Autodesk Fusion 360 part; units mm, degrees
(part 20 of 24)
  arc A286 (13.1064, 12.5222) -> (13.1064, 12.5984) centre (13.1064, 12.5603) ccw
  arc A287 (80.518, 13.5509) -> (80.518, 13.6271) centre (80.518, 13.589) ccw
  arc A288 (6.9723, 12.3063) -> (7.0485, 12.3063) centre (7.0104, 12.3063) ccw
  line L141 (7.2644, 10.2743) -> (7.6454, 10.2743)
  line L142 (13.3604, 11.7221) -> (13.3604, 11.1125)
  line L143 (6.1468, 11.1125) -> (7.0104, 11.1125)
  line L144 (6.1468, 11.7221) -> (6.1468, 11.1125)
  line L145 (7.0104, 11.1125) -> (7.0104, 11.7221)
  arc A289 (80.01, 13.4239) -> (80.01, 13.5001) centre (80.01, 13.462) ccw
  arc A290 (80.8101, 13.335) -> (80.7339, 13.335) centre (80.772, 13.335) ccw
  arc A291 (6.9723, 10.5283) -> (7.0485, 10.5283) centre (7.0104, 10.5283) ccw
  arc A292 (7.7724, 12.4714) -> (7.7724, 12.3952) centre (7.7724, 12.4333) ccw
  line L146 (7.7724, 12.4333) -> (12.5984, 12.4333)
  arc A293 (7.0104, 10.5283) -> (7.2644, 10.2743) centre (7.2644, 10.5283) ccw
  arc A294 (7.2644, 10.2362) -> (7.2644, 10.3124) centre (7.2644, 10.2743) ccw
  line L147 (7.0104, 11.7221) -> (6.1468, 11.7221)
  arc A295 (12.6253, 10.4282) -> (12.5715, 10.3744) centre (12.5984, 10.4013) ccw
  line L148 (7.2644, 12.5603) -> (7.6454, 12.5603)
  line L149 (13.1064, 10.2743) -> (12.7254, 10.2743)
  arc A296 (12.5984, 12.3952) -> (12.5984, 12.4714) centre (12.5984, 12.4333) ccw
  arc A297 (13.3985, 10.5283) -> (13.3223, 10.5283) centre (13.3604, 10.5283) ccw
  arc A298 (7.0485, 12.3063) -> (6.9723, 12.3063) centre (7.0104, 12.3063) ccw
  line L150 (12.5984, 12.4333) -> (12.7254, 12.5603)
  arc A299 (13.3985, 12.3063) -> (13.3223, 12.3063) centre (13.3604, 12.3063) ccw
  line L151 (81.5086, 25.0952) -> (81.5086, 25.7048)
  arc A300 (74.3331, 26.289) -> (74.2569, 26.289) centre (74.295, 26.289) ccw
  arc A301 (60.9869, 21.4899) -> (60.9331, 21.4361) centre (60.96, 21.463) ccw
  arc A302 (74.2569, 24.511) -> (74.3331, 24.511) centre (74.295, 24.511) ccw
  arc A303 (75.0301, 26.3891) -> (75.0839, 26.4429) centre (75.057, 26.416) ccw
  arc A304 (74.9569, 26.5699) -> (74.9031, 26.5161) centre (74.93, 26.543) ccw
  arc A305 (74.549, 26.5811) -> (74.549, 26.5049) centre (74.549, 26.543) ccw
  arc A306 (74.93, 24.2189) -> (74.93, 24.2951) centre (74.93, 24.257) ccw
  line L152 (75.057, 26.416) -> (74.93, 26.543)
  arc A307 (80.6069, 26.289) -> (80.6831, 26.289) centre (80.645, 26.289) ccw
  arc A308 (80.6831, 26.289) -> (80.6069, 26.289) centre (80.645, 26.289) ccw
  line L153 (73.4314, 25.7048) -> (73.4314, 25.0952)
  line L154 (80.645, 25.7048) -> (80.645, 25.0952)
  arc A309 (75.0839, 24.3571) -> (75.0301, 24.4109) centre (75.057, 24.384) ccw
  arc A310 (80.0369, 26.5161) -> (79.9831, 26.5699) centre (80.01, 26.543) ccw
  arc A311 (80.391, 26.5049) -> (80.391, 26.5811) centre (80.391, 26.543) ccw
  arc A312 (79.9831, 24.2301) -> (80.0369, 24.2839) centre (80.01, 24.257) ccw
  line L155 (80.391, 26.543) -> (80.01, 26.543)
  arc A313 (80.391, 26.5811) -> (80.391, 26.5049) centre (80.391, 26.543) ccw
  arc A314 (80.391, 24.2951) -> (80.391, 24.2189) centre (80.391, 24.257) ccw
  line L156 (75.057, 24.384) -> (74.93, 24.257)
  arc A315 (74.549, 24.2189) -> (74.549, 24.2951) centre (74.549, 24.257) ccw
  arc A316 (74.93, 26.5049) -> (74.93, 26.5811) centre (74.93, 26.543) ccw
  line L157 (73.4314, 25.0952) -> (74.295, 25.0952)
  line L158 (74.295, 25.0952) -> (74.295, 25.7048)
  line L159 (81.5086, 25.7048) -> (80.645, 25.7048)
  arc A317 (75.057, 26.4541) -> (75.057, 26.3779) centre (75.057, 26.416) ccw
  line L160 (80.645, 24.511) -> (80.645, 26.289)
  arc A318 (79.9099, 24.4109) -> (79.8561, 24.3571) centre (79.883, 24.384) ccw
  arc A319 (80.391, 24.257) -> (80.645, 24.511) centre (80.391, 24.511) ccw
  arc A320 (79.8561, 26.4429) -> (79.9099, 26.3891) centre (79.883, 26.416) ccw
  arc A321 (80.391, 24.2189) -> (80.391, 24.2951) centre (80.391, 24.257) ccw
  arc A322 (74.549, 26.543) -> (74.295, 26.289) centre (74.549, 26.289) ccw
  arc A323 (60.3631, 21.209) -> (60.2869, 21.209) centre (60.325, 21.209) ccw
  arc A324 (79.883, 24.3459) -> (79.883, 24.4221) centre (79.883, 24.384) ccw
  arc A325 (79.883, 26.3779) -> (79.883, 26.4541) centre (79.883, 26.416) ccw
  arc A326 (75.057, 24.4221) -> (75.057, 24.3459) centre (75.057, 24.384) ccw
  arc A327 (74.549, 24.2951) -> (74.549, 24.2189) centre (74.549, 24.257) ccw
  arc A328 (74.295, 24.511) -> (74.549, 24.257) centre (74.549, 24.511) ccw
  arc A329 (74.3331, 24.511) -> (74.2569, 24.511) centre (74.295, 24.511) ccw
  line L161 (61.087, 21.336) -> (60.96, 21.463)
  line L162 (74.549, 26.543) -> (74.93, 26.543)
  line L163 (74.549, 24.257) -> (74.93, 24.257)
  line L164 (79.883, 24.384) -> (80.01, 24.257)
  line L165 (79.883, 26.416) -> (80.01, 26.543)
  arc A330 (80.6831, 24.511) -> (80.6069, 24.511) centre (80.645, 24.511) ccw
  arc A331 (80.645, 26.289) -> (80.391, 26.543) centre (80.391, 26.289) ccw
  line L166 (74.295, 25.7048) -> (73.4314, 25.7048)
  line L167 (79.883, 24.384) -> (75.057, 24.384)
  arc A332 (80.01, 26.5811) -> (80.01, 26.5049) centre (80.01, 26.543) ccw
  arc A333 (66.7131, 19.431) -> (66.6369, 19.431) centre (66.675, 19.431) ccw
  line L168 (80.645, 25.0952) -> (81.5086, 25.0952)
  line L169 (80.391, 24.257) -> (80.01, 24.257)
  line L170 (79.883, 26.416) -> (75.057, 26.416)
  arc A334 (74.2569, 26.289) -> (74.3331, 26.289) centre (74.295, 26.289) ccw
  arc A335 (74.9031, 24.2839) -> (74.9569, 24.2301) centre (74.93, 24.257) ccw
  arc A336 (80.01, 24.2951) -> (80.01, 24.2189) centre (80.01, 24.257) ccw
  line L171 (74.295, 24.511) -> (74.295, 26.289)
  arc A337 (74.549, 26.5049) -> (74.549, 26.5811) centre (74.549, 26.543) ccw
  arc A338 (80.6069, 24.511) -> (80.6831, 24.511) centre (80.645, 24.511) ccw
  line L172 (67.5386, 20.0152) -> (67.5386, 20.6248)
  arc A339 (61.0601, 21.3091) -> (61.1139, 21.3629) centre (61.087, 21.336) ccw
  arc A340 (60.579, 19.1389) -> (60.579, 19.2151) centre (60.579, 19.177) ccw
  line L173 (65.913, 21.336) -> (61.087, 21.336)
  line L174 (60.579, 21.463) -> (60.96, 21.463)
  arc A341 (60.579, 19.2151) -> (60.579, 19.1389) centre (60.579, 19.177) ccw
  arc A342 (60.579, 21.4249) -> (60.579, 21.5011) centre (60.579, 21.463) ccw
  line L175 (66.675, 20.0152) -> (67.5386, 20.0152)
  arc A343 (66.421, 19.177) -> (66.675, 19.431) centre (66.421, 19.431) ccw
  arc A344 (60.2869, 19.431) -> (60.3631, 19.431) centre (60.325, 19.431) ccw
  arc A345 (60.96, 21.4249) -> (60.96, 21.5011) centre (60.96, 21.463) ccw
  arc A346 (66.04, 19.2151) -> (66.04, 19.1389) centre (66.04, 19.177) ccw
  arc A347 (65.913, 19.2659) -> (65.913, 19.3421) centre (65.913, 19.304) ccw
  line L176 (66.421, 19.177) -> (66.04, 19.177)
  arc A348 (60.3631, 19.431) -> (60.2869, 19.431) centre (60.325, 19.431) ccw
  line L177 (59.4614, 20.6248) -> (59.4614, 20.0152)
  arc A349 (66.675, 21.209) -> (66.421, 21.463) centre (66.421, 21.209) ccw
  line L178 (65.913, 21.336) -> (66.04, 21.463)
  arc A350 (66.04, 21.5011) -> (66.04, 21.4249) centre (66.04, 21.463) ccw
  line L179 (60.325, 20.6248) -> (59.4614, 20.6248)
  arc A351 (66.421, 21.4249) -> (66.421, 21.5011) centre (66.421, 21.463) ccw
  arc A352 (60.325, 19.431) -> (60.579, 19.177) centre (60.579, 19.431) ccw
  arc A353 (60.3631, 24.511) -> (60.2869, 24.511) centre (60.325, 24.511) ccw
  line L180 (65.913, 26.416) -> (66.04, 26.543)
  arc A354 (61.087, 19.3421) -> (61.087, 19.2659) centre (61.087, 19.304) ccw
  line L181 (60.325, 19.431) -> (60.325, 21.209)
  arc A355 (66.421, 21.5011) -> (66.421, 21.4249) centre (66.421, 21.463) ccw
  line L182 (59.4614, 20.0152) -> (60.325, 20.0152)
  line L183 (65.913, 19.304) -> (61.087, 19.304)
  arc A356 (66.04, 24.2951) -> (66.04, 24.2189) centre (66.04, 24.257) ccw
  arc A357 (66.421, 26.5049) -> (66.421, 26.5811) centre (66.421, 26.543) ccw
  line L184 (60.325, 25.7048) -> (59.4614, 25.7048)
  arc A358 (66.0669, 26.5161) -> (66.0131, 26.5699) centre (66.04, 26.543) ccw
  arc A359 (66.7131, 21.209) -> (66.6369, 21.209) centre (66.675, 21.209) ccw
  line L185 (61.087, 19.304) -> (60.96, 19.177)
  line L186 (66.675, 20.6248) -> (66.675, 20.0152)
  arc A360 (65.913, 21.2979) -> (65.913, 21.3741) centre (65.913, 21.336) ccw
  arc A361 (66.6369, 21.209) -> (66.7131, 21.209) centre (66.675, 21.209) ccw
  arc A362 (61.1139, 19.2771) -> (61.0601, 19.3309) centre (61.087, 19.304) ccw
  arc A363 (60.579, 26.5049) -> (60.579, 26.5811) centre (60.579, 26.543) ccw
  arc A364 (60.579, 21.463) -> (60.325, 21.209) centre (60.579, 21.209) ccw
  arc A365 (66.0669, 21.4361) -> (66.0131, 21.4899) centre (66.04, 21.463) ccw
  line L187 (65.913, 24.384) -> (66.04, 24.257)
  arc A366 (66.7131, 24.511) -> (66.6369, 24.511) centre (66.675, 24.511) ccw
  line L188 (60.579, 19.177) -> (60.96, 19.177)
  line L189 (66.675, 19.431) -> (66.675, 21.209)
  arc A367 (66.6369, 19.431) -> (66.7131, 19.431) centre (66.675, 19.431) ccw
  arc A368 (61.087, 21.3741) -> (61.087, 21.2979) centre (61.087, 21.336) ccw
  line L190 (66.421, 21.463) -> (66.04, 21.463)
  arc A369 (65.8861, 21.3629) -> (65.9399, 21.3091) centre (65.913, 21.336) ccw
  arc A370 (66.421, 19.1389) -> (66.421, 19.2151) centre (66.421, 19.177) ccw
  line L191 (65.913, 19.304) -> (66.04, 19.177)
  arc A371 (66.421, 19.2151) -> (66.421, 19.1389) centre (66.421, 19.177) ccw
  arc A372 (60.9331, 19.2039) -> (60.9869, 19.1501) centre (60.96, 19.177) ccw
  line L192 (67.5386, 20.6248) -> (66.675, 20.6248)
  arc A373 (66.0131, 24.2301) -> (66.0669, 24.2839) centre (66.04, 24.257) ccw
  line L193 (66.421, 26.543) -> (66.04, 26.543)
  arc A374 (66.6369, 26.289) -> (66.7131, 26.289) centre (66.675, 26.289) ccw
  arc A375 (60.96, 19.1389) -> (60.96, 19.2151) centre (60.96, 19.177) ccw
  line L194 (60.325, 20.0152) -> (60.325, 20.6248)
  arc A376 (65.9399, 19.3309) -> (65.8861, 19.2771) centre (65.913, 19.304) ccw
  arc A377 (60.2869, 21.209) -> (60.3631, 21.209) centre (60.325, 21.209) ccw
  arc A378 (60.579, 21.5011) -> (60.579, 21.4249) centre (60.579, 21.463) ccw
  arc A379 (66.0131, 19.1501) -> (66.0669, 19.2039) centre (66.04, 19.177) ccw
  line L195 (67.5386, 25.0952) -> (67.5386, 25.7048)
  line L196 (59.4614, 25.0952) -> (60.325, 25.0952)
  arc A380 (42.799, 34.1249) -> (42.799, 34.2011) centre (42.799, 34.163) ccw
  arc A381 (60.9869, 26.5699) -> (60.9331, 26.5161) centre (60.96, 26.543) ccw
  line L197 (43.307, 34.036) -> (48.133, 34.036)
  arc A382 (42.799, 31.8389) -> (42.799, 31.9151) centre (42.799, 31.877) ccw
  arc A383 (48.641, 31.877) -> (48.895, 32.131) centre (48.641, 32.131) ccw
  arc A384 (60.579, 26.5811) -> (60.579, 26.5049) centre (60.579, 26.543) ccw
  arc A385 (43.1531, 31.9039) -> (43.2069, 31.8501) centre (43.18, 31.877) ccw
  arc A386 (66.7131, 26.289) -> (66.6369, 26.289) centre (66.675, 26.289) ccw
  line L198 (42.545, 33.909) -> (42.545, 32.131)
  arc A387 (42.5831, 33.909) -> (42.5069, 33.909) centre (42.545, 33.909) ccw
  arc A388 (60.579, 26.543) -> (60.325, 26.289) centre (60.579, 26.289) ccw
  arc A389 (60.96, 24.2189) -> (60.96, 24.2951) centre (60.96, 24.257) ccw
  arc A390 (60.3631, 26.289) -> (60.2869, 26.289) centre (60.325, 26.289) ccw
  arc A391 (65.9399, 24.4109) -> (65.8861, 24.3571) centre (65.913, 24.384) ccw
  line L199 (48.133, 32.004) -> (48.26, 31.877)
  line L200 (60.325, 26.289) -> (60.325, 24.511)
  line L201 (48.641, 31.877) -> (48.26, 31.877)
  arc A392 (60.96, 26.5049) -> (60.96, 26.5811) centre (60.96, 26.543) ccw
  line L202 (61.087, 26.416) -> (65.913, 26.416)
  line L203 (61.087, 26.416) -> (60.96, 26.543)
  arc A393 (60.2869, 24.511) -> (60.3631, 24.511) centre (60.325, 24.511) ccw
  arc A394 (60.579, 24.2189) -> (60.579, 24.2951) centre (60.579, 24.257) ccw
  arc A395 (61.1139, 24.3571) -> (61.0601, 24.4109) centre (61.087, 24.384) ccw
  arc A396 (48.895, 33.909) -> (48.641, 34.163) centre (48.641, 33.909) ccw
  arc A397 (42.799, 34.163) -> (42.545, 33.909) centre (42.799, 33.909) ccw
  line L204 (61.087, 24.384) -> (60.96, 24.257)
  line L205 (67.5386, 25.7048) -> (66.675, 25.7048)
  arc A398 (60.9331, 24.2839) -> (60.9869, 24.2301) centre (60.96, 24.257) ccw
  arc A399 (61.0601, 26.3891) -> (61.1139, 26.4429) centre (61.087, 26.416) ccw
  line L206 (60.325, 25.0952) -> (60.325, 25.7048)
  arc A400 (48.8569, 33.909) -> (48.9331, 33.909) centre (48.895, 33.909) ccw
  line L207 (59.4614, 25.7048) -> (59.4614, 25.0952)
  arc A401 (60.579, 24.2951) -> (60.579, 24.2189) centre (60.579, 24.257) ccw
  line L208 (60.579, 26.543) -> (60.96, 26.543)
  arc A402 (48.641, 34.2011) -> (48.641, 34.1249) centre (48.641, 34.163) ccw
  arc A403 (66.421, 26.5811) -> (66.421, 26.5049) centre (66.421, 26.543) ccw
  arc A404 (66.675, 26.289) -> (66.421, 26.543) centre (66.421, 26.289) ccw
  arc A405 (48.9331, 32.131) -> (48.8569, 32.131) centre (48.895, 32.131) ccw
  arc A406 (48.2869, 34.1361) -> (48.2331, 34.1899) centre (48.26, 34.163) ccw
  arc A407 (65.913, 24.3459) -> (65.913, 24.4221) centre (65.913, 24.384) ccw
  arc A408 (48.641, 31.9151) -> (48.641, 31.8389) centre (48.641, 31.877) ccw
  line L209 (42.545, 33.3248) -> (41.6814, 33.3248)
  arc A409 (60.2869, 26.289) -> (60.3631, 26.289) centre (60.325, 26.289) ccw
  arc A410 (66.421, 24.2951) -> (66.421, 24.2189) centre (66.421, 24.257) ccw
  line L210 (60.579, 24.257) -> (60.96, 24.257)
  line L211 (66.675, 25.0952) -> (67.5386, 25.0952)
  line L212 (43.307, 32.004) -> (48.133, 32.004)
  arc A411 (60.325, 24.511) -> (60.579, 24.257) centre (60.579, 24.511) ccw
  arc A412 (66.421, 24.2189) -> (66.421, 24.2951) centre (66.421, 24.257) ccw
  arc A413 (61.087, 26.4541) -> (61.087, 26.3779) centre (61.087, 26.416) ccw
  line L213 (61.087, 24.384) -> (65.913, 24.384)
  arc A414 (43.307, 34.0741) -> (43.307, 33.9979) centre (43.307, 34.036) ccw
  arc A415 (66.04, 26.5811) -> (66.04, 26.5049) centre (66.04, 26.543) ccw
  arc A416 (48.26, 31.9151) -> (48.26, 31.8389) centre (48.26, 31.877) ccw
  line L214 (66.421, 24.257) -> (66.04, 24.257)
  arc A417 (61.087, 24.4221) -> (61.087, 24.3459) centre (61.087, 24.384) ccw
  line L215 (66.675, 26.289) -> (66.675, 24.511)
  arc A418 (66.6369, 24.511) -> (66.7131, 24.511) centre (66.675, 24.511) ccw
  arc A419 (66.421, 24.257) -> (66.675, 24.511) centre (66.421, 24.511) ccw
  arc A420 (65.8861, 26.4429) -> (65.9399, 26.3891) centre (65.913, 26.416) ccw
  arc A421 (65.913, 26.3779) -> (65.913, 26.4541) centre (65.913, 26.416) ccw
  line L216 (66.675, 25.7048) -> (66.675, 25.0952)
  arc A422 (43.3339, 31.9771) -> (43.2801, 32.0309) centre (43.307, 32.004) ccw
  arc A423 (48.641, 31.8389) -> (48.641, 31.9151) centre (48.641, 31.877) ccw
  line L217 (49.7586, 38.4048) -> (48.895, 38.4048)
  line L218 (48.895, 33.909) -> (48.895, 32.131)
  arc A424 (48.9331, 33.909) -> (48.8569, 33.909) centre (48.895, 33.909) ccw
  line L219 (48.895, 38.4048) -> (48.895, 37.7952)
  arc A425 (48.1599, 37.1109) -> (48.1061, 37.0571) centre (48.133, 37.084) ccw
  line L220 (49.7586, 37.7952) -> (49.7586, 38.4048)
  arc A426 (48.641, 39.2049) -> (48.641, 39.2811) centre (48.641, 39.243) ccw
  arc A427 (48.26, 34.2011) -> (48.26, 34.1249) centre (48.26, 34.163) ccw
  line L221 (42.799, 39.243) -> (43.18, 39.243)
  line L222 (43.307, 37.084) -> (43.18, 36.957)
  line L223 (49.7586, 32.7152) -> (49.7586, 33.3248)
  arc A428 (48.1599, 32.0309) -> (48.1061, 31.9771) centre (48.133, 32.004) ccw
  arc A429 (42.5831, 38.989) -> (42.5069, 38.989) centre (42.545, 38.989) ccw
  arc A430 (48.2331, 31.8501) -> (48.2869, 31.9039) centre (48.26, 31.877) ccw
  line L224 (43.307, 39.116) -> (48.133, 39.116)
  arc A431 (43.307, 37.1221) -> (43.307, 37.0459) centre (43.307, 37.084) ccw
  arc A432 (42.5069, 38.989) -> (42.5831, 38.989) centre (42.545, 38.989) ccw
  line L225 (41.6814, 37.7952) -> (42.545, 37.7952)
  line L226 (48.895, 38.989) -> (48.895, 37.211)
  arc A433 (42.545, 37.211) -> (42.799, 36.957) centre (42.799, 37.211) ccw
  line L227 (42.545, 32.7152) -> (42.545, 33.3248)
  arc A434 (42.545, 32.131) -> (42.799, 31.877) centre (42.799, 32.131) ccw
  arc A435 (48.133, 33.9979) -> (48.133, 34.0741) centre (48.133, 34.036) ccw
  line L228 (48.895, 37.7952) -> (49.7586, 37.7952)
  arc A436 (48.8569, 32.131) -> (48.9331, 32.131) centre (48.895, 32.131) ccw
  arc A437 (42.799, 39.243) -> (42.545, 38.989) centre (42.799, 38.989) ccw
  arc A438 (48.1061, 34.0629) -> (48.1599, 34.0091) centre (48.133, 34.036) ccw
  arc A439 (48.8569, 37.211) -> (48.9331, 37.211) centre (48.895, 37.211) ccw
  arc A440 (42.5069, 37.211) -> (42.5831, 37.211) centre (42.545, 37.211) ccw
  line L229 (43.307, 37.084) -> (48.133, 37.084)
  arc A441 (48.8569, 38.989) -> (48.9331, 38.989) centre (48.895, 38.989) ccw
  arc A442 (43.307, 32.0421) -> (43.307, 31.9659) centre (43.307, 32.004) ccw
  arc A443 (48.133, 39.0779) -> (48.133, 39.1541) centre (48.133, 39.116) ccw
  line L230 (48.133, 39.116) -> (48.26, 39.243)
  line L231 (48.895, 32.7152) -> (49.7586, 32.7152)
  arc A444 (43.18, 31.8389) -> (43.18, 31.9151) centre (43.18, 31.877) ccw
  arc A445 (42.799, 31.9151) -> (42.799, 31.8389) centre (42.799, 31.877) ccw
  arc A446 (42.5069, 32.131) -> (42.5831, 32.131) centre (42.545, 32.131) ccw
  arc A447 (48.133, 31.9659) -> (48.133, 32.0421) centre (48.133, 32.004) ccw
  line L232 (48.133, 37.084) -> (48.26, 36.957)
  arc A448 (48.2869, 39.2161) -> (48.2331, 39.2699) centre (48.26, 39.243) ccw
  line L233 (42.799, 31.877) -> (43.18, 31.877)
  arc A449 (43.2069, 34.1899) -> (43.1531, 34.1361) centre (43.18, 34.163) ccw
  arc A450 (43.18, 34.1249) -> (43.18, 34.2011) centre (43.18, 34.163) ccw
  arc A451 (43.18, 36.9189) -> (43.18, 36.9951) centre (43.18, 36.957) ccw
  line L234 (48.641, 34.163) -> (48.26, 34.163)
  line L235 (42.799, 34.163) -> (43.18, 34.163)
  line L236 (43.307, 34.036) -> (43.18, 34.163)
  arc A452 (42.5831, 32.131) -> (42.5069, 32.131) centre (42.545, 32.131) ccw
  line L237 (48.133, 34.036) -> (48.26, 34.163)
  line L238 (49.7586, 33.3248) -> (48.895, 33.3248)
  arc A453 (43.2801, 34.0091) -> (43.3339, 34.0629) centre (43.307, 34.036) ccw
  line L239 (41.6814, 32.7152) -> (42.545, 32.7152)
  line L240 (43.307, 32.004) -> (43.18, 31.877)
  arc A454 (42.5069, 33.909) -> (42.5831, 33.909) centre (42.545, 33.909) ccw
  arc A455 (42.799, 34.2011) -> (42.799, 34.1249) centre (42.799, 34.163) ccw
  line L241 (41.6814, 33.3248) -> (41.6814, 32.7152)
  arc A456 (48.641, 34.1249) -> (48.641, 34.2011) centre (48.641, 34.163) ccw
  line L242 (42.545, 37.7952) -> (42.545, 38.4048)
  line L243 (48.895, 33.3248) -> (48.895, 32.7152)
  arc A457 (42.799, 39.2049) -> (42.799, 39.2811) centre (42.799, 39.243) ccw
  line L244 (48.641, 40.767) -> (48.26, 40.767)
  arc A458 (43.307, 40.9321) -> (43.307, 40.8559) centre (43.307, 40.894) ccw
  arc A459 (48.641, 39.2811) -> (48.641, 39.2049) centre (48.641, 39.243) ccw
  arc A460 (48.895, 42.799) -> (48.641, 43.053) centre (48.641, 42.799) ccw
  arc A461 (48.641, 36.9951) -> (48.641, 36.9189) centre (48.641, 36.957) ccw
  line L245 (48.641, 39.243) -> (48.26, 39.243)
  arc A462 (42.799, 36.9951) -> (42.799, 36.9189) centre (42.799, 36.957) ccw
  arc A463 (42.5831, 37.211) -> (42.5069, 37.211) centre (42.545, 37.211) ccw
  arc A464 (48.895, 38.989) -> (48.641, 39.243) centre (48.641, 38.989) ccw
  line L246 (42.545, 38.989) -> (42.545, 37.211)
  arc A465 (43.1531, 36.9839) -> (43.2069, 36.9301) centre (43.18, 36.957) ccw
  arc A466 (48.9331, 38.989) -> (48.8569, 38.989) centre (48.895, 38.989) ccw
  arc A467 (48.641, 36.957) -> (48.895, 37.211) centre (48.641, 37.211) ccw
  arc A468 (48.26, 39.2811) -> (48.26, 39.2049) centre (48.26, 39.243) ccw
  arc A469 (48.9331, 37.211) -> (48.8569, 37.211) centre (48.895, 37.211) ccw
  line L247 (48.641, 36.957) -> (48.26, 36.957)
  arc A470 (48.2331, 36.9301) -> (48.2869, 36.9839) centre (48.26, 36.957) ccw
  arc A471 (43.3339, 37.0571) -> (43.2801, 37.1109) centre (43.307, 37.084) ccw
  line L248 (43.307, 40.894) -> (43.18, 40.767)
  line L249 (41.6814, 38.4048) -> (41.6814, 37.7952)
  arc A472 (42.799, 39.2811) -> (42.799, 39.2049) centre (42.799, 39.243) ccw
  arc A473 (42.5069, 42.799) -> (42.5831, 42.799) centre (42.545, 42.799) ccw
  line L250 (48.895, 41.6052) -> (49.7586, 41.6052)
  arc A474 (42.799, 40.7289) -> (42.799, 40.8051) centre (42.799, 40.767) ccw
  line L251 (43.307, 39.116) -> (43.18, 39.243)
  arc A475 (43.18, 39.2049) -> (43.18, 39.2811) centre (43.18, 39.243) ccw
  arc A476 (42.799, 36.9189) -> (42.799, 36.9951) centre (42.799, 36.957) ccw
  line L252 (42.545, 41.021) -> (42.545, 42.799)
  line L253 (42.799, 36.957) -> (43.18, 36.957)
  arc A477 (48.8569, 42.799) -> (48.9331, 42.799) centre (48.895, 42.799) ccw
  line L254 (48.133, 42.926) -> (48.26, 43.053)
  line L255 (42.545, 38.4048) -> (41.6814, 38.4048)
  arc A478 (48.1061, 39.1429) -> (48.1599, 39.0891) centre (48.133, 39.116) ccw
  arc A479 (43.2801, 42.8991) -> (43.3339, 42.9529) centre (43.307, 42.926) ccw
  arc A480 (48.1599, 40.9209) -> (48.1061, 40.8671) centre (48.133, 40.894) ccw
  line L256 (48.895, 42.2148) -> (48.895, 41.6052)
  arc A481 (43.18, 40.7289) -> (43.18, 40.8051) centre (43.18, 40.767) ccw
  arc A482 (48.133, 42.8879) -> (48.133, 42.9641) centre (48.133, 42.926) ccw
  arc A483 (48.26, 36.9951) -> (48.26, 36.9189) centre (48.26, 36.957) ccw
  line L257 (48.895, 41.021) -> (48.895, 42.799)
  arc A484 (43.307, 39.1541) -> (43.307, 39.0779) centre (43.307, 39.116) ccw
  line L258 (48.133, 40.894) -> (43.307, 40.894)
  arc A485 (43.2801, 39.0891) -> (43.3339, 39.1429) centre (43.307, 39.116) ccw
  arc A486 (43.2069, 39.2699) -> (43.1531, 39.2161) centre (43.18, 39.243) ccw
  arc A487 (48.641, 36.9189) -> (48.641, 36.9951) centre (48.641, 36.957) ccw
  arc A488 (48.133, 37.0459) -> (48.133, 37.1221) centre (48.133, 37.084) ccw
  arc A489 (48.9331, 41.021) -> (48.8569, 41.021) centre (48.895, 41.021) ccw
  line L259 (42.799, 43.053) -> (43.18, 43.053)
  arc A490 (48.2869, 43.0261) -> (48.2331, 43.0799) centre (48.26, 43.053) ccw
  arc A491 (48.641, 43.0149) -> (48.641, 43.0911) centre (48.641, 43.053) ccw
  arc A492 (28.5369, 41.021) -> (28.6131, 41.021) centre (28.575, 41.021) ccw
  line L260 (42.799, 40.767) -> (43.18, 40.767)
  line L261 (48.133, 42.926) -> (43.307, 42.926)
  arc A493 (48.26, 40.8051) -> (48.26, 40.7289) centre (48.26, 40.767) ccw
  arc A494 (48.641, 40.8051) -> (48.641, 40.7289) centre (48.641, 40.767) ccw
  arc A495 (48.1061, 42.9529) -> (48.1599, 42.8991) centre (48.133, 42.926) ccw
  arc A496 (48.641, 43.0911) -> (48.641, 43.0149) centre (48.641, 43.053) ccw
  arc A497 (42.5831, 42.799) -> (42.5069, 42.799) centre (42.545, 42.799) ccw
  arc A498 (42.799, 40.8051) -> (42.799, 40.7289) centre (42.799, 40.767) ccw
  arc A499 (43.307, 42.9641) -> (43.307, 42.8879) centre (43.307, 42.926) ccw
  arc A500 (43.18, 43.0149) -> (43.18, 43.0911) centre (43.18, 43.053) ccw
  arc A501 (48.133, 40.8559) -> (48.133, 40.9321) centre (48.133, 40.894) ccw
  arc A502 (48.26, 43.0911) -> (48.26, 43.0149) centre (48.26, 43.053) ccw
  line L262 (29.337, 42.926) -> (29.21, 43.053)
  line L263 (48.641, 43.053) -> (48.26, 43.053)
  arc A503 (29.3639, 40.8671) -> (29.3101, 40.9209) centre (29.337, 40.894) ccw
  arc A504 (43.3339, 40.8671) -> (43.2801, 40.9209) centre (43.307, 40.894) ccw
  arc A505 (29.1831, 40.7939) -> (29.2369, 40.7401) centre (29.21, 40.767) ccw
  arc A506 (34.29, 43.0911) -> (34.29, 43.0149) centre (34.29, 43.053) ccw
  arc A507 (28.829, 40.8051) -> (28.829, 40.7289) centre (28.829, 40.767) ccw
  arc A508 (42.799, 43.0911) -> (42.799, 43.0149) centre (42.799, 43.053) ccw
  arc A509 (48.2331, 40.7401) -> (48.2869, 40.7939) centre (48.26, 40.767) ccw
  line L264 (34.163, 40.894) -> (34.29, 40.767)
  arc A510 (42.799, 43.053) -> (42.545, 42.799) centre (42.799, 42.799) ccw
  arc A511 (42.5069, 41.021) -> (42.5831, 41.021) centre (42.545, 41.021) ccw
  arc A512 (42.799, 43.0149) -> (42.799, 43.0911) centre (42.799, 43.053) ccw
  line L265 (42.545, 41.6052) -> (42.545, 42.2148)
  line L266 (49.7586, 41.6052) -> (49.7586, 42.2148)
  line L267 (41.6814, 42.2148) -> (41.6814, 41.6052)
  arc A513 (43.2069, 43.0799) -> (43.1531, 43.0261) centre (43.18, 43.053) ccw
  line L268 (28.829, 43.053) -> (29.21, 43.053)
  arc A514 (29.3101, 42.8991) -> (29.3639, 42.9529) centre (29.337, 42.926) ccw
  arc A515 (43.1531, 40.7939) -> (43.2069, 40.7401) centre (43.18, 40.767) ccw
  arc A516 (34.671, 40.7289) -> (34.671, 40.8051) centre (34.671, 40.767) ccw
  line L269 (43.307, 42.926) -> (43.18, 43.053)
  line L270 (34.671, 40.767) -> (34.29, 40.767)
  arc A517 (48.9331, 42.799) -> (48.8569, 42.799) centre (48.895, 42.799) ccw
  arc A518 (42.545, 41.021) -> (42.799, 40.767) centre (42.799, 41.021) ccw
  arc A519 (34.163, 42.8879) -> (34.163, 42.9641) centre (34.163, 42.926) ccw
  arc A520 (34.671, 40.767) -> (34.925, 41.021) centre (34.671, 41.021) ccw
  line L271 (28.575, 41.021) -> (28.575, 42.799)
  arc A521 (48.8569, 41.021) -> (48.9331, 41.021) centre (48.895, 41.021) ccw
  arc A522 (48.641, 40.7289) -> (48.641, 40.8051) centre (48.641, 40.767) ccw
  arc A523 (34.163, 40.8559) -> (34.163, 40.9321) centre (34.163, 40.894) ccw
  line L272 (48.133, 40.894) -> (48.26, 40.767)
  line L273 (42.545, 42.2148) -> (41.6814, 42.2148)
  line L274 (49.7586, 42.2148) -> (48.895, 42.2148)
  arc A524 (34.9631, 41.021) -> (34.8869, 41.021) centre (34.925, 41.021) ccw
  arc A525 (34.671, 43.0149) -> (34.671, 43.0911) centre (34.671, 43.053) ccw
  arc A526 (42.5831, 41.021) -> (42.5069, 41.021) centre (42.545, 41.021) ccw
  arc A527 (34.8869, 42.799) -> (34.9631, 42.799) centre (34.925, 42.799) ccw
  arc A528 (28.575, 41.021) -> (28.829, 40.767) centre (28.829, 41.021) ccw
  arc A529 (48.641, 40.767) -> (48.895, 41.021) centre (48.641, 41.021) ccw
  line L275 (41.6814, 41.6052) -> (42.545, 41.6052)
  arc A530 (34.671, 43.0911) -> (34.671, 43.0149) centre (34.671, 43.053) ccw
  arc A531 (13.081, 16.4211) -> (13.081, 16.3449) centre (13.081, 16.383) ccw
  arc A532 (28.6131, 42.799) -> (28.5369, 42.799) centre (28.575, 42.799) ccw
  arc A533 (34.9631, 42.799) -> (34.8869, 42.799) centre (34.925, 42.799) ccw
  arc A534 (13.081, 16.3449) -> (13.081, 16.4211) centre (13.081, 16.383) ccw
  arc A535 (34.925, 42.799) -> (34.671, 43.053) centre (34.671, 42.799) ccw
  arc A536 (34.29, 40.8051) -> (34.29, 40.7289) centre (34.29, 40.767) ccw
  arc A537 (28.829, 43.053) -> (28.575, 42.799) centre (28.829, 42.799) ccw
  arc A538 (29.337, 42.9641) -> (29.337, 42.8879) centre (29.337, 42.926) ccw
  arc A539 (34.2631, 40.7401) -> (34.3169, 40.7939) centre (34.29, 40.767) ccw
  arc A540 (29.21, 43.0149) -> (29.21, 43.0911) centre (29.21, 43.053) ccw
  arc A541 (34.671, 40.8051) -> (34.671, 40.7289) centre (34.671, 40.767) ccw
  arc A542 (28.829, 43.0149) -> (28.829, 43.0911) centre (28.829, 43.053) ccw
  arc A543 (7.7739, 14.1971) -> (7.7201, 14.2509) centre (7.747, 14.224) ccw
  line L276 (13.081, 16.383) -> (12.7, 16.383)
  line L277 (28.829, 40.767) -> (29.21, 40.767)
  line L278 (27.7114, 42.2148) -> (27.7114, 41.6052)
  arc A544 (28.6131, 41.021) -> (28.5369, 41.021) centre (28.575, 41.021) ccw
  line L279 (34.925, 41.021) -> (34.925, 42.799)
  arc A545 (34.3169, 43.0261) -> (34.2631, 43.0799) centre (34.29, 43.053) ccw
  arc A546 (12.5999, 14.2509) -> (12.5461, 14.1971) centre (12.573, 14.224) ccw
  arc A547 (7.6469, 16.4099) -> (7.5931, 16.3561) centre (7.62, 16.383) ccw
  arc A548 (29.21, 40.7289) -> (29.21, 40.8051) centre (29.21, 40.767) ccw
  line L280 (34.925, 41.6052) -> (35.7886, 41.6052)
  arc A549 (12.573, 14.1859) -> (12.573, 14.2621) centre (12.573, 14.224) ccw
  line L281 (28.575, 41.6052) -> (28.575, 42.2148)
  line L282 (35.7886, 42.2148) -> (34.925, 42.2148)
  arc A550 (28.829, 43.0911) -> (28.829, 43.0149) centre (28.829, 43.053) ccw
  line L283 (27.7114, 41.6052) -> (28.575, 41.6052)
  arc A551 (13.081, 14.097) -> (13.335, 14.351) centre (13.081, 14.351) ccw
  line L284 (7.747, 16.256) -> (12.573, 16.256)
  arc A552 (7.239, 16.383) -> (6.985, 16.129) centre (7.239, 16.129) ccw
  arc A553 (12.7, 14.1351) -> (12.7, 14.0589) centre (12.7, 14.097) ccw
  line L285 (12.573, 16.256) -> (12.7, 16.383)
  line L286 (13.335, 16.129) -> (13.335, 14.351)
  line L287 (29.337, 40.894) -> (29.21, 40.767)
  arc A554 (34.1899, 40.9209) -> (34.1361, 40.8671) centre (34.163, 40.894) ccw
  arc A555 (28.829, 40.7289) -> (28.829, 40.8051) centre (28.829, 40.767) ccw
  arc A556 (13.2969, 14.351) -> (13.3731, 14.351) centre (13.335, 14.351) ccw
  line L288 (35.7886, 41.6052) -> (35.7886, 42.2148)
  line L289 (34.671, 43.053) -> (34.29, 43.053)
  arc A557 (6.9469, 16.129) -> (7.0231, 16.129) centre (6.985, 16.129) ccw
  arc A558 (12.573, 16.2179) -> (12.573, 16.2941) centre (12.573, 16.256) ccw
  arc A559 (7.0231, 14.351) -> (6.9469, 14.351) centre (6.985, 14.351) ccw
  arc A560 (29.2369, 43.0799) -> (29.1831, 43.0261) centre (29.21, 43.053) ccw
  line L290 (13.081, 14.097) -> (12.7, 14.097)
  arc A561 (7.747, 16.2941) -> (7.747, 16.2179) centre (7.747, 16.256) ccw
  arc A562 (7.239, 14.0589) -> (7.239, 14.1351) centre (7.239, 14.097) ccw
  arc A563 (34.8869, 41.021) -> (34.9631, 41.021) centre (34.925, 41.021) ccw
  line L291 (7.747, 14.224) -> (7.62, 14.097)
  line L292 (34.925, 42.2148) -> (34.925, 41.6052)
  arc A564 (13.335, 16.129) -> (13.081, 16.383) centre (13.081, 16.129) ccw
  arc A565 (28.5369, 42.799) -> (28.6131, 42.799) centre (28.575, 42.799) ccw
  line L293 (34.163, 42.926) -> (34.29, 43.053)
  line L294 (12.573, 14.224) -> (12.7, 14.097)
  line L295 (34.163, 40.894) -> (29.337, 40.894)
  arc A566 (12.6731, 14.0701) -> (12.7269, 14.1239) centre (12.7, 14.097) ccw
  line L296 (34.163, 42.926) -> (29.337, 42.926)
  line L297 (28.575, 42.2148) -> (27.7114, 42.2148)
  line L298 (7.747, 16.256) -> (7.62, 16.383)
  arc A567 (29.337, 40.9321) -> (29.337, 40.8559) centre (29.337, 40.894) ccw
  arc A568 (34.1361, 42.9529) -> (34.1899, 42.8991) centre (34.163, 42.926) ccw
  arc A569 (13.3731, 16.129) -> (13.2969, 16.129) centre (13.335, 16.129) ccw
  arc A570 (13.081, 14.1351) -> (13.081, 14.0589) centre (13.081, 14.097) ccw
  arc A571 (12.7, 16.4211) -> (12.7, 16.3449) centre (12.7, 16.383) ccw
  line L299 (6.985, 15.5448) -> (6.1214, 15.5448)
  line L300 (7.747, 14.224) -> (12.573, 14.224)
  arc A572 (12.5461, 16.2829) -> (12.5999, 16.2291) centre (12.573, 16.256) ccw
  arc A573 (13.3731, 14.351) -> (13.2969, 14.351) centre (13.335, 14.351) ccw
  arc A574 (7.239, 16.3449) -> (7.239, 16.4211) centre (7.239, 16.383) ccw
  arc A575 (7.239, 14.1351) -> (7.239, 14.0589) centre (7.239, 14.097) ccw
  line L301 (6.1214, 14.9352) -> (6.985, 14.9352)
  arc A576 (7.62, 16.3449) -> (7.62, 16.4211) centre (7.62, 16.383) ccw
  arc A577 (7.62, 14.0589) -> (7.62, 14.1351) centre (7.62, 14.097) ccw
  arc A578 (12.7269, 16.3561) -> (12.6731, 16.4099) centre (12.7, 16.383) ccw
  arc A579 (7.747, 14.2621) -> (7.747, 14.1859) centre (7.747, 14.224) ccw
  arc A580 (6.9469, 14.351) -> (7.0231, 14.351) centre (6.985, 14.351) ccw
  arc A581 (13.2969, 16.129) -> (13.3731, 16.129) centre (13.335, 16.129) ccw
  arc A582 (13.081, 14.0589) -> (13.081, 14.1351) centre (13.081, 14.097) ccw
  arc A583 (6.985, 14.351) -> (7.239, 14.097) centre (7.239, 14.351) ccw
  line L302 (7.239, 14.097) -> (7.62, 14.097)
  arc A584 (7.5931, 14.1239) -> (7.6469, 14.0701) centre (7.62, 14.097) ccw
  arc A585 (7.7201, 16.2291) -> (7.7739, 16.2829) centre (7.747, 16.256) ccw
  line L303 (13.335, 14.9352) -> (14.1986, 14.9352)
  arc A586 (21.4559, 38.2265) -> (21.971, 38.545) centre (20.3211, 40.6376) ccw
  arc A587 (19.1706, 38.1983) -> (19.1976, 38.2557) centre (19.1841, 38.227) ccw
  arc A588 (80.4672, 18.034) -> (80.5688, 18.034) centre (80.518, 18.034) ccw
  arc A589 (5.207, 29.1465) -> (5.207, 29.2735) centre (5.207, 29.21) ccw
  arc A590 (80.5688, 20.048) -> (80.4672, 20.048) centre (80.518, 20.048) ccw
  line L304 (74.4499, 6.1715) -> (74.4499, 4.1275)
  arc A591 (7.62, 26.67) -> (7.62, 24.13) centre (7.62, 25.4) ccw
  arc A592 (4.5085, 28.575) -> (4.6355, 28.575) centre (4.572, 28.575) ccw
  arc A593 (7.239, 16.4211) -> (7.239, 16.3449) centre (7.239, 16.383) ccw
  arc A594 (80.4951, 4.1275) -> (80.5967, 4.1275) centre (80.5459, 4.1275) ccw
  arc A595 (74.3991, 4.1275) -> (74.5007, 4.1275) centre (74.4499, 4.1275) ccw
  line L305 (13.335, 15.5448) -> (13.335, 14.9352)
  arc A596 (75.311, 22.1488) -> (75.311, 22.0472) centre (75.311, 22.098) ccw
  arc A597 (7.62, 18.415) -> (7.62, 32.385) centre (7.62, 25.4) ccw
  line L306 (79.629, 22.098) -> (75.311, 22.098)
  arc A598 (79.629, 15.9512) -> (79.629, 16.0528) centre (79.629, 16.002) ccw
  line L307 (75.3389, 2.0955) -> (79.6569, 2.0955)
  line L308 (80.518, 20.048) -> (80.518, 18.034)
  arc A599 (4.6355, 29.845) -> (4.5085, 29.845) centre (4.572, 29.845) ccw
  line L309 (21.971, 38.545) -> (21.971, 42.735)
  line L310 (80.5459, 6.1415) -> (80.5459, 4.1275)
  arc A600 (79.6569, 8.1407) -> (79.6569, 8.2423) centre (79.6569, 8.1915) ccw
  arc A601 (75.3389, 2.1463) -> (75.3389, 2.0447) centre (75.3389, 2.0955) ccw
  arc A602 (77.47, 17.272) -> (77.47, 20.828) centre (77.47, 19.05) ccw
  arc A603 (77.47, 20.828) -> (77.47, 17.272) centre (77.47, 19.05) ccw
  line L311 (6.985, 14.9352) -> (6.985, 15.5448)
  arc A604 (77.4979, 6.9215) -> (77.4979, 3.3655) centre (77.4979, 5.1435) ccw
  arc A605 (4.572, 30.48) -> (4.572, 27.94) centre (4.572, 29.21) ccw
  arc A606 (7.62, 24.13) -> (7.62, 26.67) centre (7.62, 25.4) ccw
  arc A607 (77.4979, 3.3655) -> (77.4979, 6.9215) centre (77.4979, 5.1435) ccw
  arc A608 (75.311, 16.0528) -> (75.311, 15.9512) centre (75.311, 16.002) ccw
  line L312 (14.1986, 15.5448) -> (13.335, 15.5448)
  arc A609 (79.6569, 2.0447) -> (79.6569, 2.1463) centre (79.6569, 2.0955) ccw
  arc A610 (74.4728, 20.078) -> (74.3712, 20.078) centre (74.422, 20.078) ccw
  arc A611 (21.9513, 42.7101) -> (21.9907, 42.7599) centre (21.971, 42.735) ccw
  arc A612 (79.629, 22.0472) -> (79.629, 22.1488) centre (79.629, 22.098) ccw
  arc A613 (4.572, 27.94) -> (4.572, 30.48) centre (4.572, 29.21) ccw
  line L313 (4.572, 28.575) -> (4.572, 29.845)
  arc A614 (20.4788, 42.044) -> (20.4153, 42.044) centre (20.4471, 42.044) ccw
  line L314 (14.1986, 14.9352) -> (14.1986, 15.5448)
  line L315 (6.985, 16.129) -> (6.985, 14.351)
  arc A615 (75.3389, 8.2423) -> (75.3389, 8.1407) centre (75.3389, 8.1915) ccw
  arc A616 (7.0231, 16.129) -> (6.9469, 16.129) centre (6.985, 16.129) ccw
  line L316 (6.1214, 15.5448) -> (6.1214, 14.9352)
  line L317 (7.239, 16.383) -> (7.62, 16.383)
  arc A617 (80.5967, 6.1415) -> (80.4951, 6.1415) centre (80.5459, 6.1415) ccw
  line L318 (75.311, 16.002) -> (79.629, 16.002)
  arc A618 (74.3712, 18.034) -> (74.4728, 18.034) centre (74.422, 18.034) ccw
  line L319 (3.937, 29.21) -> (5.207, 29.21)
  arc A619 (7.62, 32.385) -> (7.62, 18.415) centre (7.62, 25.4) ccw
  arc A620 (3.937, 29.2735) -> (3.937, 29.1465) centre (3.937, 29.21) ccw
  arc A621 (74.5007, 6.1715) -> (74.3991, 6.1715) centre (74.4499, 6.1715) ccw
  line L320 (79.6569, 8.1915) -> (75.3389, 8.1915)
  line L321 (74.422, 20.078) -> (74.422, 18.034)
  arc A622 (21.445, 43.0936) -> (21.4186, 43.0358) centre (21.4318, 43.0647) ccw
  arc A623 (20.4788, 39.504) -> (20.4153, 39.504) centre (20.4471, 39.504) ccw
  arc A624 (20.4153, 39.236) -> (20.4788, 39.236) centre (20.4471, 39.236) ccw
  arc A625 (20.4153, 41.776) -> (20.4788, 41.776) centre (20.4471, 41.776) ccw
  arc A626 (22.0027, 42.735) -> (21.9393, 42.735) centre (21.971, 42.735) ccw
  line L322 (20.447, 42.044) -> (20.447, 41.776)
  arc A627 (21.9393, 38.545) -> (22.0027, 38.545) centre (21.971, 38.545) ccw
  arc A628 (19.1841, 43.053) -> (19.1841, 38.227) centre (20.3201, 40.64) ccw
  arc A629 (21.9907, 38.5201) -> (21.9513, 38.5699) centre (21.971, 38.545) ccw
  arc A630 (21.971, 42.735) -> (21.4318, 43.0647) centre (20.321, 40.6423) ccw
  arc A631 (21.4424, 38.2552) -> (21.4694, 38.1978) centre (21.4559, 38.2265) ccw
  arc A632 (19.1976, 43.0243) -> (19.1706, 43.0817) centre (19.1841, 43.053) ccw
  line L323 (20.447, 39.504) -> (20.447, 39.236)
  line L324 (75.311, 22.098) -> (74.422, 22.098)
  line L325 (74.422, 22.098) -> (74.422, 20.078)
  line L326 (74.422, 18.034) -> (74.422, 16.002)
  line L327 (74.422, 16.002) -> (75.311, 16.002)
  line L328 (79.629, 16.002) -> (80.518, 16.002)
  line L329 (80.518, 16.002) -> (80.518, 18.034)
  line L330 (79.629, 22.098) -> (80.518, 22.098)
  line L331 (80.518, 22.098) -> (80.518, 20.048)
  line L332 (75.3389, 8.1915) -> (74.4499, 8.1915)
  line L333 (74.4499, 8.1915) -> (74.4499, 6.1715)
  line L334 (74.4499, 4.1275) -> (74.4499, 2.0955)
  line L335 (74.4499, 2.0955) -> (75.3389, 2.0955)
  line L336 (79.6569, 2.0955) -> (80.5459, 2.0955)
  line L337 (80.5459, 2.0955) -> (80.5459, 4.1275)
  line L338 (79.6569, 8.1915) -> (80.5459, 8.1915)
  line L339 (80.5459, 8.1915) -> (80.5459, 6.1415)
  arc A633 (21.4318, 43.0647) -> (19.1841, 43.053) centre (20.3205, 40.6413) ccw
  arc A634 (19.1841, 38.227) -> (21.4559, 38.2265) centre (20.3205, 40.641) ccw
  arc A635 (14.8844, 6.2992) -> (13.0344, 6.283) centre (13.97, 5.0798) ccw
  arc A636 (13.0344, 3.877) -> (14.8558, 3.8399) centre (13.97, 5.0802) ccw
  arc A637 (5.9817, 6.2865) -> (4.1317, 6.2703) centre (5.0673, 5.0671) ccw
  arc A638 (4.1317, 3.8643) -> (5.9531, 3.8272) centre (5.0673, 5.0675) ccw
  constraint coincident A596.centre L306.end
  constraint perpendicular L321 L324
  constraint coincident A610.centre L321.start
  constraint perpendicular L324 L325
  constraint coincident A618.centre L321.end
  constraint perpendicular L318 L326
  constraint coincident A608.centre L318.start
  constraint perpendicular L326 L327
  constraint coincident A598.centre L318.end
  constraint perpendicular L308 L328
  constraint coincident A588.centre L308.end
  constraint perpendicular L328 L329
  constraint coincident L306.start A612.centre
  constraint perpendicular L308 L330
  constraint coincident A590.centre L308.start
  constraint perpendicular L330 L331
  constraint coincident A615.centre L320.end
  constraint perpendicular L304 L332
  constraint coincident L304.start A621.centre
  constraint perpendicular L332 L333
  constraint coincident L304.end A595.centre
  constraint perpendicular L307 L334
  constraint coincident L307.start A601.centre
  constraint perpendicular L334 L335
  constraint coincident L307.end A609.centre
  constraint perpendicular L310 L336
  constraint coincident A594.centre L310.end
  constraint perpendicular L336 L337
  constraint coincident A600.centre L320.start
  constraint perpendicular L310 L338
  constraint coincident L310.start A617.centre
  constraint perpendicular L320 L339
  constraint coincident A622.centre A630.end
  constraint tangent A630 A633
  constraint tangent A628 A634
  constraint tangent A222 A635
  constraint tangent A238 A636
  constraint tangent A171 A638
  constraint tangent A242 A637